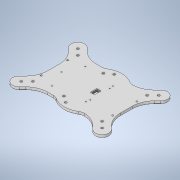
# Autodesk Inventor part: BaseTop_v1
Saved by Autodesk Inventor 2020.3 (Build 243373000, 373)
## iProperties
Created: 2021-03-02
Part Number: BaseTop_v1
Material: Generic
Document SubType Name: Modeling
Designer: sanyi
Density: 1 g/cm^3
Appearance: Default
Author: sanyi
Autodesk Inventor part; units mm, degrees
ref_plane "YZ Plane" through (0, 0, 0) normal (1, 0, 0) x (0, 1, 0)
ref_plane "XZ Plane" through (0, 0, 0) normal (0, 1, 0) x (-1, 0, 0)
ref_plane "XY Plane" through (0, 0, 0) normal (0, 0, 1) x (1, 0, 0)
sketch "Sketch1" plane through (0, 0, 0) normal (0, 1, 0) x (-1, 0, 0)
  line L0 (0, 114.5572) -> (0, -115.3318) construction
  line L1 (119.9398, 0) -> (-136.2559, 0) construction
  line L2 (67.5, 45) -> (32.9932, 45) construction
  line L3 (-67.5, 45) -> (-67.5, 10.4932) construction
  line L4 (-67.5, -45) -> (-19.7, -45) construction
  line L5 (67.5, -45) -> (67.5, -10.4932) construction
  line L6 (66.7599, -35.4918) -> (84.1548, -52.8866) construction
  line L7 (84.1548, -52.8866) -> (75.3866, -61.6548) construction
  line L8 (75.3866, -61.6548) -> (57.9918, -44.2599) construction
  line L9 (57.9918, -44.2599) -> (62.3759, -39.8759) construction
  line L10 (66.7599, 35.4918) -> (84.1548, 52.8866) construction
  line L11 (84.1548, 52.8866) -> (75.3866, 61.6548) construction
  line L12 (75.3866, 61.6548) -> (57.9918, 44.2599) construction
  line L13 (57.9918, 44.2599) -> (62.3759, 39.8759) construction
  line L14 (-57.9918, 44.2599) -> (-75.3866, 61.6548) construction
  line L15 (-75.3866, 61.6548) -> (-84.1548, 52.8866) construction
  line L16 (-84.1548, 52.8866) -> (-66.7599, 35.4918) construction
  line L17 (-66.7599, 35.4918) -> (-57.9918, 44.2599) construction
  line L18 (-57.9918, -44.2599) -> (-75.3866, -61.6548) construction
  line L19 (-75.3866, -61.6548) -> (-84.1548, -52.8866) construction
  line L20 (-84.1548, -52.8866) -> (-66.7599, -35.4918) construction
  line L21 (-66.7599, -35.4918) -> (-57.9918, -44.2599) construction
  line L22 (75.4574, 44.1892) -> (66.6892, 52.9574) construction
  line L23 (70.5783, 56.8464) -> (79.3464, 48.0783) construction
  circle A0 centre (74.9624, 52.4624) radius 4.35 construction
  line L24 (75.4574, -44.1892) -> (66.6892, -52.9574) construction
  line L25 (79.3464, -48.0783) -> (70.5783, -56.8464) construction
  circle A1 centre (74.9624, -52.4624) radius 4.35 construction
  line L26 (-66.6892, 52.9574) -> (-75.4574, 44.1892) construction
  line L27 (-70.5783, 56.8464) -> (-79.3464, 48.0783) construction
  circle A2 centre (-74.9624, 52.4624) radius 4.35 construction
  line L28 (-75.4574, -44.1892) -> (-66.6892, -52.9574) construction
  line L29 (-79.3464, -48.0783) -> (-70.5783, -56.8464) construction
  circle A3 centre (-74.9624, -52.4624) radius 4.35 construction
  line L30 (6.8, 51.2) -> (-17.8, 51.2) construction
  line L31 (-17.8, 51.2) -> (-17.8, 38.8) construction
  line L32 (-17.8, 38.8) -> (6.8, 38.8) construction
  line L33 (6.8, 38.8) -> (6.8, 51.2) construction
  line L34 (6.8, -38.8) -> (-17.8, -38.8) construction
  line L35 (-17.8, -38.8) -> (-17.8, -51.2) construction
  line L36 (-17.8, -51.2) -> (6.8, -51.2) construction
  line L37 (6.8, -51.2) -> (6.8, -38.8) construction
  line L38 (6.8, 45) -> (-17.8, 45) construction
  line L39 (-5.5, 51.2) -> (-5.5, 38.8) construction
  line L40 (0, 51.2) -> (0, 38.8) construction
  line L41 (6.8, -45) -> (-17.8, -45) construction
  line L42 (-5.5, -38.8) -> (-5.5, -51.2) construction
  line L43 (0, -38.8) -> (0, -51.2) construction
  circle A4 centre (0, 45) radius 4.35 construction
  circle A5 centre (0, -45) radius 4.35 construction
  line L44 (20, 30) -> (20, -30) construction
  line L45 (8.8, 57.2) -> (-19.8, 57.2)
  line L46 (8.8, -57.2) -> (-19.8, -57.2)
  line L47 (8.8, 57.2) -> (8.8, 45) construction
  line L48 (-19.8, 57.2) -> (-19.8, 45) construction
  line L49 (8.8, -57.2) -> (8.8, -45) construction
  line L50 (-19.8, -57.2) -> (-19.8, -45) construction
  line L51 (68.3156, 63.069) -> (62.4466, 57.2)
  line L52 (85.569, 45.8156) -> (79.7, 39.9466)
  line L53 (66.6892, 52.9574) -> (62.4466, 57.2) construction
  line L54 (75.4574, 44.1892) -> (79.7, 39.9466) construction
  arc A6 (85.569, 45.8156) -> (68.3156, 63.069) centre (76.9423, 54.4423) ccw
  line L55 (-62.4466, 57.2) -> (-68.3156, 63.069)
  line L56 (-85.569, 45.8156) -> (-79.7, 39.9466)
  line L57 (-62.4466, 57.2) -> (-66.6892, 52.9574) construction
  line L58 (-79.7, 39.9466) -> (-75.4574, 44.1892) construction
  arc A7 (-68.3156, 63.069) -> (-85.569, 45.8156) centre (-76.9423, 54.4423) ccw
  line L59 (75.4574, -44.1892) -> (79.7, -39.9466) construction
  line L60 (79.7, -39.9466) -> (85.569, -45.8156)
  line L61 (66.6892, -52.9574) -> (62.4466, -57.2) construction
  line L62 (62.4466, -57.2) -> (68.3156, -63.069)
  arc A8 (68.3156, -63.069) -> (85.569, -45.8156) centre (76.9423, -54.4423) ccw
  line L63 (-75.4574, -44.1892) -> (-79.7, -39.9466) construction
  line L64 (-66.6892, -52.9574) -> (-62.4466, -57.2) construction
  line L65 (-62.4466, -57.2) -> (-68.3156, -63.069)
  line L66 (-79.7, -39.9466) -> (-85.569, -45.8156)
  arc A9 (-85.569, -45.8156) -> (-68.3156, -63.069) centre (-76.9423, -54.4423) ccw
  arc A10 (23.5363, -45) -> (8.8, -57.2) centre (23.5363, -60) ccw
  arc A11 (62.4466, -57.2) -> (32.9932, -45) centre (32.9932, -86.6534) ccw
  arc A12 (67.5, -10.4932) -> (79.7, -39.9466) centre (109.1534, -10.4932) ccw
  arc A13 (79.7, 39.9466) -> (67.5, 10.4932) centre (109.1534, 10.4932) ccw
  arc A14 (32.9932, 45) -> (62.4466, 57.2) centre (32.9932, 86.6534) ccw
  arc A15 (8.8, 57.2) -> (23.5363, 45) centre (23.5363, 60) ccw
  arc A16 (-67.5, 10.4932) -> (-79.7, 39.9466) centre (-109.1534, 10.4932) ccw
  arc A17 (-79.7, -39.9466) -> (-67.5, -10.4932) centre (-109.1534, -10.4932) ccw
  line L67 (74.9624, -52.4624) -> (-74.9624, -52.4624) construction
  line L68 (-74.9624, 52.4624) -> (74.9624, 52.4624) construction
  line L69 (-62.4466, 57.2) -> (-62.4466, 45) construction
  line L70 (-62.4466, -57.2) -> (-62.4466, -45) construction
  arc A18 (-19.8, -57.2) -> (-34.5363, -45) centre (-34.5363, -60) ccw
  arc A19 (-32.9932, -45) -> (-62.4466, -57.2) centre (-32.9932, -86.6534) ccw
  line L71 (75.3866, 61.6548) -> (78.2151, 64.4832) construction
  line L72 (78.2151, 64.4832) -> (86.9832, 55.7151) construction
  line L73 (86.9832, 55.7151) -> (84.1548, 52.8866) construction
  line L74 (81.1142, 58.6142) -> (61.0324, 38.5324) construction
  line L75 (61.0324, -38.5324) -> (81.1142, -58.6142) construction
  line L76 (-81.1142, 58.6142) -> (-61.0324, 38.5324) construction
  line L77 (-81.1142, -58.6142) -> (-61.0324, -38.5324) construction
  line L78 (76.9423, 54.4423) -> (79.7707, 57.2707) construction
  line L79 (76.9423, -54.4423) -> (79.7707, -57.2707) construction
  line L80 (-76.9423, -54.4423) -> (-79.7707, -57.2707) construction
  line L81 (-76.9423, 54.4423) -> (-79.7707, 57.2707) construction
  line L82 (-19.7, 45) -> (-67.5, 45) construction
  line L83 (8.7, 45) -> (-19.7, 45) construction
  line L84 (8.7, -45) -> (23.5363, -45) construction
  line L85 (-19.7, -45) -> (8.7, -45) construction
  line L86 (81.9627, 55.0787) -> (77.1544, 50.2704) construction
  line L87 (72.7704, -54.6544) -> (77.5787, -59.4627) construction
  line L88 (0, -48.1) -> (6.8, -48.1) construction
  line L89 (-77.1544, -50.2704) -> (-81.9627, -55.0787) construction
  line L90 (-77.5787, 59.4627) -> (-72.7704, 54.6544) construction
  line L91 (0, 48.1) -> (6.8, 48.1) construction
  line L92 (32.9932, 45) -> (23.5363, 45)
  line L93 (23.5363, 45) -> (8.7, 45) construction
  line L94 (32.9932, -45) -> (67.5, -45) construction
  line L95 (23.5363, -45) -> (32.9932, -45)
  line L96 (67.5, -10.4932) -> (67.5, 10.4932)
  line L97 (67.5, 10.4932) -> (67.5, 45) construction
  line L98 (-67.5, 10.4932) -> (-67.5, -10.4932)
  line L99 (-67.5, -10.4932) -> (-67.5, -45) construction
  line L100 (39.5, 31) -> (39.5, -31)
  line L101 (39.5, -31) -> (-17.5, -25)
  line L102 (-17.5, -25) -> (-17.5, 25)
  line L103 (-17.5, 25) -> (39.5, 31)
  line L104 (52.8, 0) -> (-18.5, 18)
  line L105 (-18.5, 18) -> (-18.5, -18)
  line L106 (-18.5, -18) -> (52.8, 0)
  line L107 (17.5, 30) -> (17.5, -30) construction
  line L108 (-18.5, 10) -> (-40.2, 10) construction
  line L109 (-40.2, 10) -> (-40.2, -10) construction
  line L110 (-40.2, -10) -> (-18.5, -10) construction
  line L111 (-17.5, 20) -> (-52.2, 20) construction
  line L112 (-52.2, 20) -> (-52.2, -20) construction
  line L113 (-52.2, -20) -> (-17.5, -20) construction
  line L114 (-34.5363, -45) -> (-32.9932, -45)
  arc A20 (-34.5363, 45) -> (-19.8, 57.2) centre (-34.5363, 60) ccw
  arc A21 (-62.4466, 57.2) -> (-32.9932, 45) centre (-32.9932, 86.6534) ccw
  line L115 (-32.9932, 45) -> (-34.5363, 45)
  line L116 (66.3287, 39.6329) -> (62.212, 43.7497) construction
  line L117 (62.3759, 39.8759) -> (66.7599, 35.4918) construction
  line L118 (65.7725, -40.1891) -> (63.0378, -42.9239) construction
  line L119 (62.3759, -39.8759) -> (66.7599, -35.4918) construction
  line L120 (-62.4668, -43.4949) -> (-65.8513, -40.1104) construction
  line L121 (-62.8091, 43.1525) -> (-65.1909, 40.7708) construction
  circle A22 centre (11.7808, 36.6) radius 6 construction
  line L122 (6.8, 38.8) -> (6.8, 32.8) construction
  line L123 (6.8, 32.8) -> (-17.8, 32.8) construction
  line L124 (-17.8, 32.8) -> (-17.8, 38.8) construction
  line L125 (10.5333, 30.7311) -> (0.8, 32.8) construction
  circle A23 centre (11.7808, -36.6) radius 6 construction
  line L126 (6.8, -38.8) -> (6.8, -32.8) construction
  line L127 (6.8, -32.8) -> (-17.8, -32.8) construction
  line L128 (-17.8, -32.8) -> (-17.8, -38.8) construction
  line L129 (10.5333, -30.7311) -> (0.8, -32.8) construction
  line L130 (15.6366, -36.6) -> (7.7217, -36.6) construction
  line L131 (14.2436, 36.6) -> (7.7217, 36.6) construction
  line L132 (65.3457, 34.0776) -> (56.5776, 42.8457) construction
  line L133 (65.3457, -34.0776) -> (56.5776, -42.8457) construction
  line L134 (-56.5776, -42.8457) -> (-65.3457, -34.0776)
  line L135 (-56.5776, 42.8457) -> (-65.3457, 34.0776)
  line L136 (-7.5, -6) -> (-13.5, -6)
  line L137 (-13.5, -6) -> (-13.5, 6)
  line L138 (-13.5, 6) -> (-7.5, 6)
  line L139 (-7.5, 6) -> (-7.5, -6)
  line L140 (-64.5, -22.5) -> (-64.5, 22.5)
  line L141 (77.5, -12.5) -> (77.5, 12.5)
  line L142 (77.5, 12.5) -> (67.5, 29.8205)
  line L143 (67.5, 29.8205) -> (67.5, 10.4932)
  line L144 (67.5, -10.4932) -> (67.5, -29.8205)
  line L145 (67.5, -29.8205) -> (77.5, -12.5)
  line L146 (77.5, -12.5) -> (73.5, -11.4282) construction
  line L147 (73.5, -11.4282) -> (73.5, 11.4282) construction
  line L148 (73.5, 11.4282) -> (77.5, 12.5) construction
  line L149 (73.5, 11.4282) -> (66, 24.4186) construction
  line L150 (73.5, -11.4282) -> (66, -24.4186) construction
  line L151 (64.5, -22.5) -> (64.5, 22.5)
  point P0 (0, 0)
  point P1 (65.0291, 0)
  point P2 (55, 0)
  point P3 (-62.3759, 39.8759)
  point P4 (-62.3759, -39.8759)
  point P5 (0, 45)
  point P6 (-33.9576, -45.0112)
  point P7 (-58.7319, -45)
  point P8 (-58.7319, 45)
  point P9 (64.2308, 41.7308)
  point P10 (64.2308, -41.7308)
  point P11 (-64.2308, -41.7308)
  point P12 (-64.2308, 41.7308)
  point P13 (-33.9576, 45.0112)
  point P14 (60.9617, 38.4617)
  point P15 (60.9617, -38.4617)
  point P16 (-60.9617, -38.4617)
  point P17 (-60.9617, 38.4617)
  dimension "d154" = 12
  dimension "d0" = 135
  dimension "d4" = 24.6
  dimension "d5" = 12.4
  dimension "d9" = 8.7
  dimension "d10" = 135
  dimension "d12" = 6
  dimension "d13" = 2
  dimension "d14" = 2
  dimension "d16" = 20
  dimension "d23" = 6
  dimension "d29" = 135
  dimension "d32" = 15
  dimension "d33" = 4
  dimension "d34" = 28.4
  dimension "d38" = 4
  dimension "d40" = 6.8
  dimension "d60" = 90
  dimension "d61" = 135
  dimension "d70" = 135
  dimension "d113" = 22
  dimension "d114" = 35
  dimension "d115" = 25
  dimension "d116" = 31
  dimension "d117" = 35.3
  dimension "d118" = 36
  dimension "d119" = 18
  dimension "d120" = 17.5
  dimension "d121" = 10
  dimension "d122" = 20
  dimension "d123" = 93
  dimension "d124" = 91.7
  dimension "d157" = 6
  dimension "d158" = 12
  dimension "d159" = 6
  dimension "d160" = 3.8
  dimension "d161" = 2
  dimension "d162" = 2
  dimension "d163" = 2
  dimension "d164" = 2
  dimension "d165" = 6
  dimension "d166" = 12
  dimension "d167" = 5
  dimension "d169" = 3
  dimension "d170" = 45
  dimension "d178" = 30
  dimension "d179" = 25
  dimension "d180" = 10
  dimension "d182" = 4
  dimension "d183" = 15
  constraints: 302 end point, 95 point on line, 73 parallel, 70 perpendicular, 56 tangent, 36 midpoint, 34 equal length, 32 point on circle, 24 symmetric about line, 22 centre point, 18 coincident, 17 horizontal, 14 collinear, 8 equal radius, 4 vertical, 41 other
  measures "d0" angle of L3 L16
  measures "d4" distance between parallel lines of L11 L13
  measures "d5" distance between parallel lines of L10 L12
  measures "d9" diameter of A0
  measures "d10" angle of L6 L5
  measures "d12" distance between parallel lines of L30 L45
  measures "d13" distance between parallel lines of L33 L47
  measures "d14" distance between parallel lines of L37 L49
  measures "d16" distance between parallel lines of L0 L44
  measures "d23" distance between parallel lines of L52 L10
  measures "d29" distance between parallel lines of L3 L5
  measures "d32" radius of A15
  measures "d33" distance between parallel lines of L72 L11
  measures "d34" distance of L74.start L74.end
  measures "d38" distance of L78.start L78.end
  measures "d40" distance between parallel lines of L11 L23
  measures "d60" distance between parallel lines of L2 L84
  measures "d61" angle of L97 L10
  measures "d70" angle of L99 L20
  measures "d113" distance between parallel lines of L107 L100
  measures "d114" distance between parallel lines of L102 L107
  measures "d115" distance from line of L101.end L1
  measures "d116" distance from line of L1 L100.end
  measures "d117" distance from line of L107 L104.start
  measures "d118" distance between parallel lines of L105 L107
  measures "d119" distance from line of L1 L105.end
  measures "d120" distance between parallel lines of L0 L107
  measures "d121" distance between parallel lines of L1 L110
  measures "d122" distance between parallel lines of L1 L113
  measures "d123" distance from line of L104.start L109
  measures "d124" distance between parallel lines of L100 L112
  measures "d157" distance between parallel lines of L32 L123
  measures "d158" angle of L125 L123
  measures "d159" distance of L122.end L125.end
  measures "d160" distance between parallel lines of L123 L131
  measures "d161" distance between parallel lines of L117 L132
  measures "d162" distance between parallel lines of L9 L133
  measures "d163" distance between parallel lines of L134 L21
  measures "d164" distance between parallel lines of L17 L135
  measures "d165" distance of L137.end L138.end
  measures "d166" distance of L136.end L137.end
  measures "d167" distance between parallel lines of L105 L137
  measures "d169" distance between parallel lines of L98 L140
  measures "d170" distance of L140.start L140.end
  measures "d178" angle of L5 L145
  measures "d179" distance of L141.start L141.end
  measures "d180" distance between parallel lines of L96 L141
  measures "d182" distance between parallel lines of L141 L147
  measures "d183" distance of L146.end L150.end
extrude "Extrusion12" add sketch "Sketch1" along normal blind 5 contours A21 L115 A20 | A18 L114 A19 | A15 L92 A14 L51 A6 L52 A13 L142 L143 L96 L144 L145 A12 L60 A8 L62 A11 L95 A10 L46 A18 A19 L65 A9 L66 A17 L98 A16 L56 A7 L55 A21 A20 L45 | A13 L143 L142 | A12 L145 L144 | L100 L104 L102 L103 | L104 L106 L100 | L100 L106 L102 L104 | L100 L101 L102 L106 | L102 L106 L105 L104
hole "Hole2" at (0, 0, 45) at (74.9624, 0, 52.4624) at (74.9624, 0, -52.4624) at (0, 0, -45) at (-74.9624, 0, -52.4624) at (-74.9624, 0, 52.4624) at (-64.2308, 0, 41.7308) at (-64.2308, 0, -41.7308) at (64.2308, 0, -41.7308) at (64.2308, 0, 41.7308) at (-11.7808, 0, 36.6) at (-11.7808, 0, -36.6) direction (0, 1, 0) diameter 4.2 depth 5 countersink diameter 8.3 countersink angle 90
fillet "Fillet10" radius 40 4 edges at (-8.8, 2.5, 57.2) (-8.8, 2.5, -57.2) (19.8, 2.5, -57.2) (19.8, 2.5, 57.2)
hole "Hole3" at (-39.5, 0, 31) at (-39.5, 0, -31) at (-52.8, 0, 0) at (18.5, 0, -18) at (17.5, 0, -25) at (18.5, 0, 18) at (17.5, 0, 25) direction (0, 1, 0) diameter 1.9 depth 5
fillet "Fillet15" radius 0.5 30 edges at (65.3811, 0, 60.1345) (85.569, 0, 63.069) (82.6345, 0, 42.8811) (70.6707, 0, 26.4333) (67.5, 0, 0) (70.6707, 0, -26.4333) (82.6345, 0, -42.8811) (85.569, 0, -63.069) (65.3811, 0, -60.1345) (49.3777, 0, -48.3578) (49.3777, 0, 48.3578) (30.1411, 0, 45.6584) (-19.4187, 0, 45.5762) (-28.2648, 0, 45) (-48.9333, 0, 48.1707) (-65.3811, 0, 60.1345) (-85.569, 0, 63.069) (-82.6345, 0, 42.8811) (-70.6707, 0, 26.4333) (-67.5, 0, 0) (-70.6707, 0, -26.4333) (-82.6345, 0, -42.8811) (-85.569, 0, -63.069) (-65.3811, 0, -60.1345) (-48.9333, 0, -48.1707) (-28.2648, 0, -45) (-19.4187, 0, -45.5762) (5.5, 0, -53.2893) (30.1411, 0, -45.6584) (5.5, 0, 53.2893)
fillet "Fillet15" radius 1 4 edges at (7.5, 0, 0) (7.5, 5, 0) (13.5, 5, 0) (13.5, 0, 0)
hole "Hole4" at (64.5, 0, -22.5) at (64.5, 0, 22.5) at (-66, 0, -24.4186) at (-66, 0, 24.4186) direction (0, 1, 0) diameter 3 depth 5 countersink diameter 6.3 countersink angle 90
body "Solid6"
